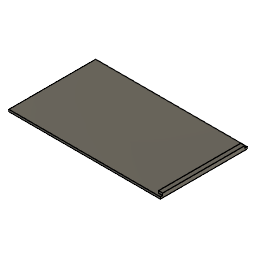
Control board - top plate v1 (Autodesk Fusion 360 design; units mm, degrees)
Autodesk Fusion 360 part; units mm, degrees
sketch "Sketch1" plane through (0, 0, 0) normal (0, 0, 1) x (1, 0, 0)
  line L0 (0, 30) -> (72.9, 30)
  line L1 (72.9, 30) -> (72.9, -11.8)
  line L2 (72.9, -11.8) -> (0, -11.8)
  line L3 (0, -11.8) -> (0, 30)
  dimension "d1" = 72.9
  dimension "d2" = 41.8
  constraint horizontal L0
  constraint vertical L1
  constraint horizontal L2
  constraint vertical L3
  measures "d1" distance of L0.start L0.end
  measures "d2" distance of L0.end L1.end
extrude "Extrude1" add sketch "Sketch1" along normal blind 1
sketch "Sketch2" plane through (0, 0, 1) normal (0, 0, 1) x (-1, 0, 0)
  line L0 (0, 11.8) -> (-72.9, 11.8)
  line L1 (-72.9, 11.8) -> (-72.9, -30)
  line L2 (-72.9, -30) -> (0, -30)
  line L3 (0, -30) -> (0, 11.8)
  line L4 (0, -9.1) -> (-72.9, -9.1) construction
  line L5 (-72.9, -28.9) -> (-70.9, -28.9)
  line L6 (-70.9, -28.9) -> (-70.9, 10.7)
  line L7 (-70.9, 10.7) -> (-72.9, 10.7)
  line L8 (-72.9, 10.7) -> (-72.9, -28.9)
  dimension "d5" = 39.6
  dimension "d6" = 2
  constraint midpoint L3 L4.start
  constraint midpoint L1 L4.end
  constraint horizontal L5
  constraint vertical L6
  constraint horizontal L7
  constraint vertical L8
  constraint coincident L1 L5.start
  constraint symmetric L4 L5 L7
  measures "d5" distance of L5.end L6.end
  measures "d6" distance of L5.start L5.end
extrude "Extrude2" add sketch "Sketch2" along normal blind 1 contours L1 L5 L6 L7 L8
